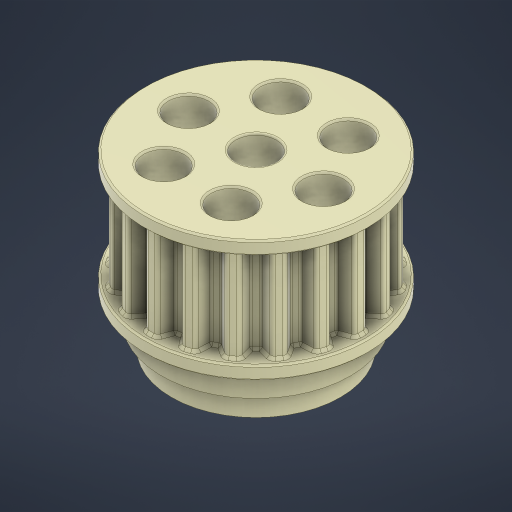
# Autodesk Inventor part: Pulley_Joint1
Saved by Autodesk Inventor 2023 (Build 270158000, 158)
## iProperties
Created: 2023-02-16
Part Number: Pulley_Joint1
Material: ABS Plastic
Document SubType Name: Modeling
Designer: dzw04
Density: 1.06 g/cm^3
Appearance: Smooth - Ash
Author: dzw04
Autodesk Inventor part; units mm, degrees
ref_plane "YZ Plane" through (0, 0, 0) normal (1, 0, 0) x (0, 1, 0)
ref_plane "XZ Plane" through (0, 0, 0) normal (0, 1, 0) x (-1, 0, 0)
ref_plane "XY Plane" through (0, 0, 0) normal (0, 0, 1) x (1, 0, 0)
sketch "Sketch1" plane through (0, 0, 0) normal (0, 1, 0) x (-1, 0, 0)
  circle A0 centre (0, 0) radius 12.5
  dimension "d0" = 25
  constraints: 1 centre point, 1 coincident
  measures "d0" diameter of A0
extrude "Extrusion1" add sketch "Sketch1" along normal blind 3.5
sketch "Sketch2" plane through (0, 3.5, 0) normal (0, 1, 0) x (1, 0, 0)
  circle A0 centre (0, 0) radius 10
  circle A1 centre (-10, 0) radius 1.5
  circle A2 centre (-5, -8.6603) radius 1.5
  circle A3 centre (5, -8.6603) radius 1.5
  circle A4 centre (10, 0) radius 1.5
  circle A5 centre (5, 8.6603) radius 1.5
  circle A6 centre (-5, 8.6603) radius 1.5
  dimension "d3" = 20
  dimension "d4" = 3
  dimension "d7" = 360
  constraints: 6 centre point, 1 coincident, 1 horizontal alignment, 15 other
  measures "d4" diameter of A1
extrude "Extrusion2" cut sketch "Sketch2" against normal through all contours A0 A4 | A0 A4 | A5 A0 | A0 A5 | A3 A0 | A0 A3 | A6 A0 | A0 A6 | A2 A0 | A0 A2 | A1 A0 | A0 A1
sketch "Sketch3" plane through (0, 0, 0) normal (0, -1, 0) x (1, 0, 0)
  line L0 (0, -5.7158) -> (-4.95, -2.8579)
  line L1 (-4.95, -2.8579) -> (-4.95, 2.8579)
  line L2 (-4.95, 2.8579) -> (0, 5.7158)
  line L3 (0, 5.7158) -> (4.95, 2.8579)
  line L4 (4.95, 2.8579) -> (4.95, -2.8579)
  line L5 (4.95, -2.8579) -> (0, -5.7158)
  point P0 (0, 0)
  point P1 (0, 0)
  dimension "d11" = 4.95
  constraints: 12 end point, 1 coincident, 13 other
  measures "d11" distance from line of L5 point (0, 0)
extrude "Extrusion3" add sketch "Sketch3" along normal blind 1.75
chamfer "Chamfer1" distance 1 angle 45 6 edges at (4.95, 0, 0) (2.475, 0, 4.2868) (2.475, 0, -4.2868) (-2.475, 0, -4.2868) (-4.95, 0, 0) (-2.475, 0, 4.2868)
sketch "Sketch4" plane through (0, 3.5, 0) normal (0, 1, 0) x (1, 0, 0)
  circle A0 centre (0, 0) radius 14
  circle A1 centre (5, 8.6603) radius 1.5 projected
  circle A2 centre (-5, -8.6603) radius 1.5 projected
  circle A3 centre (-5, 8.6603) radius 1.5 projected
  circle A4 centre (10, 0) radius 1.5 projected
  circle A5 centre (5, -8.6603) radius 1.5 projected
  circle A6 centre (-10, 0) radius 1.5 projected
  circle A7 centre (0, 0) radius 12.5 projected
  dimension "d17" = 28
  constraints: 1 centre point, 1 coincident
  measures "d17" diameter of A0
extrude "Extrusion4" add sketch "Sketch4" along normal blind 6 contours A0 | A7
sketch "Sketch5" plane through (0, 9.5, 0) normal (0, 1, 0) x (1, 0, 0)
  circle A0 centre (0, 0) radius 16.5
  circle A1 centre (0, 0) radius 14
  dimension "d20" = 33
  dimension "d21" = 28
  constraints: 2 centre point, 2 coincident
  measures "d20" diameter of A0
  measures "d21" diameter of A1
extrude "Extrusion5" add sketch "Sketch5" against normal blind 2
sketch "Sketch6" plane through (0, 9.5, 0) normal (0, 1, 0) x (1, 0, 0)
  arc A0 (-1.7917, 13.431) -> (-2.4464, 13.3273) centre (0, 0) ccw
  arc A1 (-2.8316, 13.4718) -> (-2.4464, 13.3273) centre (-2.5186, 13.7208) ccw
  line L0 (-2.8316, 13.4718) -> (-3.774, 14.6565)
  arc A2 (-3.774, 14.6565) -> (-4.4144, 14.8581) centre (-4.2435, 14.2829) ccw
  arc A3 (-4.4144, 14.8581) -> (-5.162, 14.6152) centre (0, 0) ccw
  arc A4 (-5.162, 14.6152) -> (-5.5616, 14.0756) centre (-4.9622, 14.0494) ccw
  line L1 (-5.5616, 14.0756) -> (-5.6277, 12.5633)
  arc A5 (-5.8545, 12.22) -> (-5.6277, 12.5633) centre (-6.0273, 12.5807) ccw
  arc A6 (-5.8545, 12.22) -> (-6.445, 11.9191) centre (0, 0) ccw
  arc A7 (-6.856, 11.9374) -> (-6.445, 11.9191) centre (-6.6353, 12.2709) ccw
  line L2 (-6.856, 11.9374) -> (-8.1183, 12.7729)
  arc A8 (-8.1183, 12.7729) -> (-8.7898, 12.7668) centre (-8.4495, 12.2726) ccw
  arc A9 (-8.7898, 12.7668) -> (-9.4257, 12.3047) centre (0, 0) ccw
  arc A10 (-9.4257, 12.3047) -> (-9.639, 11.668) centre (-9.0609, 11.8284) ccw
  line L3 (-9.639, 11.668) -> (-9.2345, 10.2093)
  arc A11 (-9.3441, 9.8128) -> (-9.2345, 10.2093) centre (-9.6199, 10.1024) ccw
  arc A12 (-9.3441, 9.8128) -> (-9.8128, 9.3441) centre (0, 0) ccw
  arc A13 (-10.2093, 9.2345) -> (-9.8128, 9.3441) centre (-10.1024, 9.6199) ccw
  line L4 (-10.2093, 9.2345) -> (-11.668, 9.639)
  arc A14 (-11.668, 9.639) -> (-12.3047, 9.4257) centre (-11.8284, 9.0609) ccw
  arc A15 (-12.3047, 9.4257) -> (-12.7668, 8.7898) centre (0, 0) ccw
  arc A16 (-12.7668, 8.7898) -> (-12.7729, 8.1183) centre (-12.2726, 8.4495) ccw
  line L5 (-12.7729, 8.1183) -> (-11.9374, 6.856)
  arc A17 (-11.9191, 6.445) -> (-11.9374, 6.856) centre (-12.2709, 6.6353) ccw
  arc A18 (-11.9191, 6.445) -> (-12.22, 5.8545) centre (0, 0) ccw
  arc A19 (-12.5633, 5.6277) -> (-12.22, 5.8545) centre (-12.5807, 6.0273) ccw
  line L6 (-12.5633, 5.6277) -> (-14.0756, 5.5616)
  arc A20 (-14.0756, 5.5616) -> (-14.6152, 5.162) centre (-14.0494, 4.9622) ccw
  arc A21 (-14.6152, 5.162) -> (-14.8581, 4.4144) centre (0, 0) ccw
  arc A22 (-14.8581, 4.4144) -> (-14.6565, 3.774) centre (-14.2829, 4.2435) ccw
  line L7 (-14.6565, 3.774) -> (-13.4718, 2.8316)
  arc A23 (-13.3273, 2.4464) -> (-13.4718, 2.8316) centre (-13.7208, 2.5186) ccw
  arc A24 (-13.3273, 2.4464) -> (-13.431, 1.7917) centre (0, 0) ccw
  arc A25 (-13.6874, 1.47) -> (-13.431, 1.7917) centre (-13.8275, 1.8446) ccw
  line L8 (-13.6874, 1.47) -> (-15.1053, 0.9398)
  arc A26 (-15.1053, 0.9398) -> (-15.495, 0.393) centre (-14.8952, 0.3778) ccw
  arc A27 (-15.495, 0.393) -> (-15.495, -0.393) centre (0, 0) ccw
  arc A28 (-15.495, -0.393) -> (-15.1053, -0.9398) centre (-14.8952, -0.3778) ccw
  line L9 (-15.1053, -0.9398) -> (-13.6874, -1.47)
  arc A29 (-13.431, -1.7917) -> (-13.6874, -1.47) centre (-13.8275, -1.8446) ccw
  arc A30 (-13.431, -1.7917) -> (-13.3273, -2.4464) centre (0, 0) ccw
  arc A31 (-13.4718, -2.8316) -> (-13.3273, -2.4464) centre (-13.7208, -2.5186) ccw
  line L10 (-13.4718, -2.8316) -> (-14.6565, -3.774)
  arc A32 (-14.6565, -3.774) -> (-14.8581, -4.4144) centre (-14.2829, -4.2435) ccw
  arc A33 (-14.8581, -4.4144) -> (-14.6152, -5.162) centre (0, 0) ccw
  arc A34 (-14.6152, -5.162) -> (-14.0756, -5.5616) centre (-14.0494, -4.9622) ccw
  line L11 (-14.0756, -5.5616) -> (-12.5633, -5.6277)
  arc A35 (-12.22, -5.8545) -> (-12.5633, -5.6277) centre (-12.5807, -6.0273) ccw
  arc A36 (-12.22, -5.8545) -> (-11.9191, -6.445) centre (0, 0) ccw
  arc A37 (-11.9374, -6.856) -> (-11.9191, -6.445) centre (-12.2709, -6.6353) ccw
  line L12 (-11.9374, -6.856) -> (-12.7729, -8.1183)
  arc A38 (-12.7729, -8.1183) -> (-12.7668, -8.7898) centre (-12.2726, -8.4495) ccw
  arc A39 (-12.7668, -8.7898) -> (-12.3047, -9.4257) centre (0, 0) ccw
  arc A40 (-12.3047, -9.4257) -> (-11.668, -9.639) centre (-11.8284, -9.0609) ccw
  line L13 (-11.668, -9.639) -> (-10.2093, -9.2345)
  arc A41 (-9.8128, -9.3441) -> (-10.2093, -9.2345) centre (-10.1024, -9.6199) ccw
  arc A42 (-9.8128, -9.3441) -> (-9.3441, -9.8128) centre (0, 0) ccw
  arc A43 (-9.2345, -10.2093) -> (-9.3441, -9.8128) centre (-9.6199, -10.1024) ccw
  line L14 (-9.2345, -10.2093) -> (-9.639, -11.668)
  arc A44 (-9.639, -11.668) -> (-9.4257, -12.3047) centre (-9.0609, -11.8284) ccw
  arc A45 (-9.4257, -12.3047) -> (-8.7898, -12.7668) centre (0, 0) ccw
  arc A46 (-8.7898, -12.7668) -> (-8.1183, -12.7729) centre (-8.4495, -12.2726) ccw
  line L15 (-8.1183, -12.7729) -> (-6.856, -11.9374)
  arc A47 (-6.445, -11.9191) -> (-6.856, -11.9374) centre (-6.6353, -12.2709) ccw
  arc A48 (-6.445, -11.9191) -> (-5.8545, -12.22) centre (0, 0) ccw
  arc A49 (-5.6277, -12.5633) -> (-5.8545, -12.22) centre (-6.0273, -12.5807) ccw
  line L16 (-5.6277, -12.5633) -> (-5.5616, -14.0756)
  arc A50 (-5.5616, -14.0756) -> (-5.162, -14.6152) centre (-4.9622, -14.0494) ccw
  arc A51 (-5.162, -14.6152) -> (-4.4144, -14.8581) centre (0, 0) ccw
  arc A52 (-4.4144, -14.8581) -> (-3.774, -14.6565) centre (-4.2435, -14.2829) ccw
  line L17 (-3.774, -14.6565) -> (-2.8316, -13.4718)
  arc A53 (-2.4464, -13.3273) -> (-2.8316, -13.4718) centre (-2.5186, -13.7208) ccw
  arc A54 (-2.4464, -13.3273) -> (-1.7917, -13.431) centre (0, 0) ccw
  arc A55 (-1.47, -13.6874) -> (-1.7917, -13.431) centre (-1.8446, -13.8275) ccw
  line L18 (-1.47, -13.6874) -> (-0.9398, -15.1053)
  arc A56 (-0.9398, -15.1053) -> (-0.393, -15.495) centre (-0.3778, -14.8952) ccw
  arc A57 (-0.393, -15.495) -> (0.393, -15.495) centre (0, 0) ccw
  arc A58 (0.393, -15.495) -> (0.9398, -15.1053) centre (0.3778, -14.8952) ccw
  line L19 (0.9398, -15.1053) -> (1.47, -13.6874)
  arc A59 (1.7917, -13.431) -> (1.47, -13.6874) centre (1.8446, -13.8275) ccw
  arc A60 (1.7917, -13.431) -> (2.4464, -13.3273) centre (0, 0) ccw
  arc A61 (2.8316, -13.4718) -> (2.4464, -13.3273) centre (2.5186, -13.7208) ccw
  line L20 (2.8316, -13.4718) -> (3.774, -14.6565)
  arc A62 (3.774, -14.6565) -> (4.4144, -14.8581) centre (4.2435, -14.2829) ccw
  arc A63 (4.4144, -14.8581) -> (5.162, -14.6152) centre (0, 0) ccw
  arc A64 (5.162, -14.6152) -> (5.5616, -14.0756) centre (4.9622, -14.0494) ccw
  line L21 (5.5616, -14.0756) -> (5.6277, -12.5633)
  arc A65 (5.8545, -12.22) -> (5.6277, -12.5633) centre (6.0273, -12.5807) ccw
  arc A66 (5.8545, -12.22) -> (6.445, -11.9191) centre (0, 0) ccw
  arc A67 (6.856, -11.9374) -> (6.445, -11.9191) centre (6.6353, -12.2709) ccw
  line L22 (6.856, -11.9374) -> (8.1183, -12.7729)
  arc A68 (8.1183, -12.7729) -> (8.7898, -12.7668) centre (8.4495, -12.2726) ccw
  arc A69 (8.7898, -12.7668) -> (9.4257, -12.3047) centre (0, 0) ccw
  arc A70 (9.4257, -12.3047) -> (9.639, -11.668) centre (9.0609, -11.8284) ccw
  line L23 (9.639, -11.668) -> (9.2345, -10.2093)
  arc A71 (9.3441, -9.8128) -> (9.2345, -10.2093) centre (9.6199, -10.1024) ccw
  arc A72 (9.3441, -9.8128) -> (9.8128, -9.3441) centre (0, 0) ccw
  arc A73 (10.2093, -9.2345) -> (9.8128, -9.3441) centre (10.1024, -9.6199) ccw
  line L24 (10.2093, -9.2345) -> (11.668, -9.639)
  arc A74 (11.668, -9.639) -> (12.3047, -9.4257) centre (11.8284, -9.0609) ccw
  arc A75 (12.3047, -9.4257) -> (12.7668, -8.7898) centre (0, 0) ccw
  arc A76 (12.7668, -8.7898) -> (12.7729, -8.1183) centre (12.2726, -8.4495) ccw
  line L25 (12.7729, -8.1183) -> (11.9374, -6.856)
  arc A77 (11.9191, -6.445) -> (11.9374, -6.856) centre (12.2709, -6.6353) ccw
  arc A78 (11.9191, -6.445) -> (12.22, -5.8545) centre (0, 0) ccw
  arc A79 (12.5633, -5.6277) -> (12.22, -5.8545) centre (12.5807, -6.0273) ccw
  line L26 (12.5633, -5.6277) -> (14.0756, -5.5616)
  arc A80 (14.0756, -5.5616) -> (14.6152, -5.162) centre (14.0494, -4.9622) ccw
  arc A81 (14.6152, -5.162) -> (14.8581, -4.4144) centre (0, 0) ccw
  arc A82 (14.8581, -4.4144) -> (14.6565, -3.774) centre (14.2829, -4.2435) ccw
  line L27 (14.6565, -3.774) -> (13.4718, -2.8316)
  arc A83 (13.3273, -2.4464) -> (13.4718, -2.8316) centre (13.7208, -2.5186) ccw
  arc A84 (13.3273, -2.4464) -> (13.431, -1.7917) centre (0, 0) ccw
  arc A85 (13.6874, -1.47) -> (13.431, -1.7917) centre (13.8275, -1.8446) ccw
  line L28 (13.6874, -1.47) -> (15.1053, -0.9398)
  arc A86 (15.1053, -0.9398) -> (15.495, -0.393) centre (14.8952, -0.3778) ccw
  arc A87 (15.495, -0.393) -> (15.495, 0.393) centre (0, 0) ccw
  arc A88 (15.495, 0.393) -> (15.1053, 0.9398) centre (14.8952, 0.3778) ccw
  line L29 (15.1053, 0.9398) -> (13.6874, 1.47)
  arc A89 (13.431, 1.7917) -> (13.6874, 1.47) centre (13.8275, 1.8446) ccw
  arc A90 (13.431, 1.7917) -> (13.3273, 2.4464) centre (0, 0) ccw
  arc A91 (13.4718, 2.8316) -> (13.3273, 2.4464) centre (13.7208, 2.5186) ccw
  line L30 (13.4718, 2.8316) -> (14.6565, 3.774)
  arc A92 (14.6565, 3.774) -> (14.8581, 4.4144) centre (14.2829, 4.2435) ccw
  arc A93 (14.8581, 4.4144) -> (14.6152, 5.162) centre (0, 0) ccw
  arc A94 (14.6152, 5.162) -> (14.0756, 5.5616) centre (14.0494, 4.9622) ccw
  line L31 (14.0756, 5.5616) -> (12.5633, 5.6277)
  arc A95 (12.22, 5.8545) -> (12.5633, 5.6277) centre (12.5807, 6.0273) ccw
  arc A96 (12.22, 5.8545) -> (11.9191, 6.445) centre (0, 0) ccw
  arc A97 (11.9374, 6.856) -> (11.9191, 6.445) centre (12.2709, 6.6353) ccw
  line L32 (11.9374, 6.856) -> (12.7729, 8.1183)
  arc A98 (12.7729, 8.1183) -> (12.7668, 8.7898) centre (12.2726, 8.4495) ccw
  arc A99 (12.7668, 8.7898) -> (12.3047, 9.4257) centre (0, 0) ccw
  arc A100 (12.3047, 9.4257) -> (11.668, 9.639) centre (11.8284, 9.0609) ccw
  line L33 (11.668, 9.639) -> (10.2093, 9.2345)
  arc A101 (9.8128, 9.3441) -> (10.2093, 9.2345) centre (10.1024, 9.6199) ccw
  arc A102 (9.8128, 9.3441) -> (9.3441, 9.8128) centre (0, 0) ccw
  arc A103 (9.2345, 10.2093) -> (9.3441, 9.8128) centre (9.6199, 10.1024) ccw
  line L34 (9.2345, 10.2093) -> (9.639, 11.668)
  arc A104 (9.639, 11.668) -> (9.4257, 12.3047) centre (9.0609, 11.8284) ccw
  arc A105 (9.4257, 12.3047) -> (8.7898, 12.7668) centre (0, 0) ccw
  arc A106 (8.7898, 12.7668) -> (8.1183, 12.7729) centre (8.4495, 12.2726) ccw
  line L35 (8.1183, 12.7729) -> (6.856, 11.9374)
  arc A107 (6.445, 11.9191) -> (6.856, 11.9374) centre (6.6353, 12.2709) ccw
  arc A108 (6.445, 11.9191) -> (5.8545, 12.22) centre (0, 0) ccw
  arc A109 (5.6277, 12.5633) -> (5.8545, 12.22) centre (6.0273, 12.5807) ccw
  line L36 (5.6277, 12.5633) -> (5.5616, 14.0756)
  arc A110 (5.5616, 14.0756) -> (5.162, 14.6152) centre (4.9622, 14.0494) ccw
  arc A111 (5.162, 14.6152) -> (4.4144, 14.8581) centre (0, 0) ccw
  arc A112 (4.4144, 14.8581) -> (3.774, 14.6565) centre (4.2435, 14.2829) ccw
  line L37 (3.774, 14.6565) -> (2.8316, 13.4718)
  arc A113 (2.4464, 13.3273) -> (2.8316, 13.4718) centre (2.5186, 13.7208) ccw
  arc A114 (2.4464, 13.3273) -> (1.7917, 13.431) centre (0, 0) ccw
  arc A115 (1.47, 13.6874) -> (1.7917, 13.431) centre (1.8446, 13.8275) ccw
  line L38 (1.47, 13.6874) -> (0.9398, 15.1053)
  arc A116 (0.9398, 15.1053) -> (0.393, 15.495) centre (0.3778, 14.8952) ccw
  arc A117 (0.393, 15.495) -> (-0.393, 15.495) centre (0, 0) ccw
  arc A118 (-0.393, 15.495) -> (-0.9398, 15.1053) centre (-0.3778, 14.8952) ccw
  line L39 (-0.9398, 15.1053) -> (-1.47, 13.6874)
  arc A119 (-1.7917, 13.431) -> (-1.47, 13.6874) centre (-1.8446, 13.8275) ccw
  circle A120 centre (0, 0) radius 17.75
  circle A121 centre (0, 0) radius 16.5 projected
  circle A122 centre (-10, 0) radius 1.5 projected
  circle A123 centre (5, -8.6603) radius 1.5 projected
  circle A124 centre (10, 0) radius 1.5 projected
  circle A125 centre (-5, 8.6603) radius 1.5 projected
  circle A126 centre (-5, -8.6603) radius 1.5 projected
  circle A127 centre (5, 8.6603) radius 1.5 projected
  point P0 (1.47, 13.6874)
  point P1 (0.393, 15.495)
  point P2 (-0.393, 15.495)
  point P3 (-0.9398, 15.1053)
  point P4 (-1.7917, 13.431)
  point P5 (-2.4464, 13.3273)
  point P6 (-2.8316, 13.4718)
  point P7 (-4.4144, 14.8581)
  point P8 (-5.162, 14.6152)
  point P9 (-5.5616, 14.0756)
  point P10 (-5.8545, 12.22)
  point P11 (-6.445, 11.9191)
  point P12 (-6.856, 11.9374)
  point P13 (-8.7898, 12.7668)
  point P14 (-9.4257, 12.3047)
  point P15 (-9.3441, 9.8128)
  point P16 (-9.8128, 9.3441)
  point P17 (-10.2093, 9.2345)
  point P18 (-12.3047, 9.4257)
  point P19 (-12.7668, 8.7898)
  point P20 (-12.7729, 8.1183)
  point P21 (-11.9191, 6.445)
  point P22 (-12.22, 5.8545)
  point P23 (-12.5633, 5.6277)
  point P24 (-14.8581, 4.4144)
  point P25 (-14.6565, 3.774)
  point P26 (-13.3273, 2.4464)
  point P27 (-13.431, 1.7917)
  point P28 (-13.6874, 1.47)
  point P29 (-15.495, 0.393)
  point P30 (-15.495, -0.393)
  point P31 (-15.1053, -0.9398)
  point P32 (-13.3273, -2.4464)
  point P33 (-13.4718, -2.8316)
  point P34 (-14.8581, -4.4144)
  point P35 (-14.6152, -5.162)
  point P36 (-14.0756, -5.5616)
  point P37 (-12.22, -5.8545)
  point P38 (-11.9191, -6.445)
  point P39 (-12.7668, -8.7898)
  point P40 (-12.3047, -9.4257)
  point P41 (-9.8128, -9.3441)
  point P42 (-9.3441, -9.8128)
  point P43 (-9.2345, -10.2093)
  point P44 (-9.4257, -12.3047)
  point P45 (-8.7898, -12.7668)
  point P46 (-6.445, -11.9191)
  point P47 (-5.8545, -12.22)
  point P48 (-5.162, -14.6152)
  point P49 (-4.4144, -14.8581)
  point P50 (-2.4464, -13.3273)
  point P51 (-1.7917, -13.431)
  point P52 (-1.47, -13.6874)
  point P53 (-0.393, -15.495)
  point P54 (0.393, -15.495)
  point P55 (0.9398, -15.1053)
  point P56 (1.7917, -13.431)
  point P57 (2.4464, -13.3273)
  point P58 (2.8316, -13.4718)
  point P59 (4.4144, -14.8581)
  point P60 (5.162, -14.6152)
  point P61 (5.8545, -12.22)
  point P62 (6.445, -11.9191)
  point P63 (6.856, -11.9374)
  point P64 (8.7898, -12.7668)
  point P65 (9.4257, -12.3047)
  point P66 (9.3441, -9.8128)
  point P67 (9.8128, -9.3441)
  point P68 (10.2093, -9.2345)
  point P69 (12.3047, -9.4257)
  point P70 (12.7668, -8.7898)
  point P71 (12.7729, -8.1183)
  point P72 (11.9191, -6.445)
  point P73 (12.22, -5.8545)
  point P74 (12.5633, -5.6277)
  point P75 (14.6152, -5.162)
  point P76 (14.8581, -4.4144)
  point P77 (14.6565, -3.774)
  point P78 (13.3273, -2.4464)
  point P79 (13.431, -1.7917)
  point P80 (13.6874, -1.47)
  point P81 (15.495, -0.393)
  point P82 (15.495, 0.393)
  point P83 (15.1053, 0.9398)
  point P84 (13.3273, 2.4464)
  point P85 (13.4718, 2.8316)
  point P86 (14.8581, 4.4144)
  point P87 (14.6152, 5.162)
  point P88 (14.0756, 5.5616)
  point P89 (12.22, 5.8545)
  point P90 (11.9191, 6.445)
  point P91 (11.9374, 6.856)
  point P92 (12.7668, 8.7898)
  point P93 (12.3047, 9.4257)
  point P94 (9.8128, 9.3441)
  point P95 (9.3441, 9.8128)
  point P96 (9.2345, 10.2093)
  point P97 (9.4257, 12.3047)
  point P98 (8.7898, 12.7668)
  point P99 (8.1183, 12.7729)
  point P100 (6.445, 11.9191)
  point P101 (5.8545, 12.22)
  point P102 (5.6277, 12.5633)
  point P103 (5.162, 14.6152)
  point P104 (4.4144, 14.8581)
  point P105 (3.774, 14.6565)
  point P106 (2.4464, 13.3273)
  point P107 (1.7917, 13.431)
  constraints: 240 point on circle, 121 centre point, 80 end point
extrude "Extrusion6" add sketch "Sketch6" along normal blind 14 contours A119 L39 A118 A117 A116 L38 A115 A114 A113 L37 A112 A111 A110 L36 A109 A108 A107 L35 A106 A105 A104 L34 A103 A102 A101 L33 A100 A99 A98 L32 A97 A96 A95 L31 A94 A93 A92 L30 A91 A90 A89 L29 A88 A87 A86 L28 A85 A84 A83 L27 A82 A81 A80 L26 A79 A78 A77 L25 A76 A75 A74 L24 A73 A72 A71 L23 A70 A69 A68 L22 A67 A66 A65 L21 A64 A63 A62 L20 A61 A60 A59 L19 A58 A57 A56 L18 A55 A54 A53 L17 A52 A51 A50 L16 A49 A48 A47 L15 A46 A45 A44 L14 A43 A42 A41 L13 A40 A39 A38 L12 A37 A36 A35 L11 A34 A33 A32 L10 A31 A30 A29 L9 A28 A27 A26 L8 A25 A24 A23 L7 A22 A21 A20 L6 A19 A18 A17 L5 A16 A15 A14 L4 A13 A12 A11 L3 A10 A9 A8 L2 A7 A6 A5 L1 A4 A3 A2 L0 A1 A0
sketch "Sketch7" plane through (0, 23.5, 0) normal (0, 1, 0) x (1, 0, 0)
  circle A0 centre (0, 0) radius 16.5
  arc A1 (0.9398, 15.1053) -> (0.393, 15.495) centre (0.3778, 14.8952) ccw projected
  arc A2 (0.393, 15.495) -> (-0.393, 15.495) centre (0, 0) ccw projected
  arc A3 (-0.393, 15.495) -> (-0.9398, 15.1053) centre (-0.3778, 14.8952) ccw projected
  line L0 (-0.9398, 15.1053) -> (-1.47, 13.6874) projected
  arc A4 (-1.7917, 13.431) -> (-1.47, 13.6874) centre (-1.8446, 13.8275) ccw projected
  arc A5 (-1.7917, 13.431) -> (-2.4464, 13.3273) centre (0, 0) ccw projected
  arc A6 (-2.8316, 13.4718) -> (-2.4464, 13.3273) centre (-2.5186, 13.7208) ccw projected
  line L1 (-2.8316, 13.4718) -> (-3.774, 14.6565) projected
  arc A7 (-3.774, 14.6565) -> (-4.4144, 14.8581) centre (-4.2435, 14.2829) ccw projected
  arc A8 (-4.4144, 14.8581) -> (-5.162, 14.6152) centre (0, 0) ccw projected
  arc A9 (-5.162, 14.6152) -> (-5.5616, 14.0756) centre (-4.9622, 14.0494) ccw projected
  line L2 (-5.5616, 14.0756) -> (-5.6277, 12.5633) projected
  arc A10 (-5.8545, 12.22) -> (-5.6277, 12.5633) centre (-6.0273, 12.5807) ccw projected
  arc A11 (-5.8545, 12.22) -> (-6.445, 11.9191) centre (0, 0) ccw projected
  arc A12 (-6.856, 11.9374) -> (-6.445, 11.9191) centre (-6.6353, 12.2709) ccw projected
  line L3 (-6.856, 11.9374) -> (-8.1183, 12.7729) projected
  arc A13 (-8.1183, 12.7729) -> (-8.7898, 12.7668) centre (-8.4495, 12.2726) ccw projected
  arc A14 (-8.7898, 12.7668) -> (-9.4257, 12.3047) centre (0, 0) ccw projected
  arc A15 (-9.4257, 12.3047) -> (-9.639, 11.668) centre (-9.0609, 11.8284) ccw projected
  line L4 (-9.639, 11.668) -> (-9.2345, 10.2093) projected
  arc A16 (-9.3441, 9.8128) -> (-9.2345, 10.2093) centre (-9.6199, 10.1024) ccw projected
  arc A17 (-9.3441, 9.8128) -> (-9.8128, 9.3441) centre (0, 0) ccw projected
  arc A18 (-10.2093, 9.2345) -> (-9.8128, 9.3441) centre (-10.1024, 9.6199) ccw projected
  line L5 (-10.2093, 9.2345) -> (-11.668, 9.639) projected
  arc A19 (-11.668, 9.639) -> (-12.3047, 9.4257) centre (-11.8284, 9.0609) ccw projected
  arc A20 (-12.3047, 9.4257) -> (-12.7668, 8.7898) centre (0, 0) ccw projected
  arc A21 (-12.7668, 8.7898) -> (-12.7729, 8.1183) centre (-12.2726, 8.4495) ccw projected
  line L6 (-12.7729, 8.1183) -> (-11.9374, 6.856) projected
  arc A22 (-11.9191, 6.445) -> (-11.9374, 6.856) centre (-12.2709, 6.6353) ccw projected
  arc A23 (-11.9191, 6.445) -> (-12.22, 5.8545) centre (0, 0) ccw projected
  arc A24 (-12.5633, 5.6277) -> (-12.22, 5.8545) centre (-12.5807, 6.0273) ccw projected
  line L7 (-12.5633, 5.6277) -> (-14.0756, 5.5616) projected
  arc A25 (-14.0756, 5.5616) -> (-14.6152, 5.162) centre (-14.0494, 4.9622) ccw projected
  arc A26 (-14.6152, 5.162) -> (-14.8581, 4.4144) centre (0, 0) ccw projected
  arc A27 (-14.8581, 4.4144) -> (-14.6565, 3.774) centre (-14.2829, 4.2435) ccw projected
  line L8 (-14.6565, 3.774) -> (-13.4718, 2.8316) projected
  arc A28 (-13.3273, 2.4464) -> (-13.4718, 2.8316) centre (-13.7208, 2.5186) ccw projected
  arc A29 (-13.3273, 2.4464) -> (-13.431, 1.7917) centre (0, 0) ccw projected
  arc A30 (-13.6874, 1.47) -> (-13.431, 1.7917) centre (-13.8275, 1.8446) ccw projected
  line L9 (-13.6874, 1.47) -> (-15.1053, 0.9398) projected
  arc A31 (-15.1053, 0.9398) -> (-15.495, 0.393) centre (-14.8952, 0.3778) ccw projected
  arc A32 (-15.495, 0.393) -> (-15.495, -0.393) centre (0, 0) ccw projected
  arc A33 (-15.495, -0.393) -> (-15.1053, -0.9398) centre (-14.8952, -0.3778) ccw projected
  line L10 (-15.1053, -0.9398) -> (-13.6874, -1.47) projected
  arc A34 (-13.431, -1.7917) -> (-13.6874, -1.47) centre (-13.8275, -1.8446) ccw projected
  arc A35 (-13.431, -1.7917) -> (-13.3273, -2.4464) centre (0, 0) ccw projected
  arc A36 (-13.4718, -2.8316) -> (-13.3273, -2.4464) centre (-13.7208, -2.5186) ccw projected
  line L11 (-13.4718, -2.8316) -> (-14.6565, -3.774) projected
  arc A37 (-14.6565, -3.774) -> (-14.8581, -4.4144) centre (-14.2829, -4.2435) ccw projected
  arc A38 (-14.8581, -4.4144) -> (-14.6152, -5.162) centre (0, 0) ccw projected
  arc A39 (-14.6152, -5.162) -> (-14.0756, -5.5616) centre (-14.0494, -4.9622) ccw projected
  line L12 (-14.0756, -5.5616) -> (-12.5633, -5.6277) projected
  arc A40 (-12.22, -5.8545) -> (-12.5633, -5.6277) centre (-12.5807, -6.0273) ccw projected
  arc A41 (-12.22, -5.8545) -> (-11.9191, -6.445) centre (0, 0) ccw projected
  arc A42 (-11.9374, -6.856) -> (-11.9191, -6.445) centre (-12.2709, -6.6353) ccw projected
  line L13 (-11.9374, -6.856) -> (-12.7729, -8.1183) projected
  arc A43 (-12.7729, -8.1183) -> (-12.7668, -8.7898) centre (-12.2726, -8.4495) ccw projected
  arc A44 (-12.7668, -8.7898) -> (-12.3047, -9.4257) centre (0, 0) ccw projected
  arc A45 (-12.3047, -9.4257) -> (-11.668, -9.639) centre (-11.8284, -9.0609) ccw projected
  line L14 (-11.668, -9.639) -> (-10.2093, -9.2345) projected
  arc A46 (-9.8128, -9.3441) -> (-10.2093, -9.2345) centre (-10.1024, -9.6199) ccw projected
  arc A47 (-9.8128, -9.3441) -> (-9.3441, -9.8128) centre (0, 0) ccw projected
  arc A48 (-9.2345, -10.2093) -> (-9.3441, -9.8128) centre (-9.6199, -10.1024) ccw projected
  line L15 (-9.2345, -10.2093) -> (-9.639, -11.668) projected
  arc A49 (-9.639, -11.668) -> (-9.4257, -12.3047) centre (-9.0609, -11.8284) ccw projected
  arc A50 (-9.4257, -12.3047) -> (-8.7898, -12.7668) centre (0, 0) ccw projected
  arc A51 (-8.7898, -12.7668) -> (-8.1183, -12.7729) centre (-8.4495, -12.2726) ccw projected
  line L16 (-8.1183, -12.7729) -> (-6.856, -11.9374) projected
  arc A52 (-6.445, -11.9191) -> (-6.856, -11.9374) centre (-6.6353, -12.2709) ccw projected
  arc A53 (-6.445, -11.9191) -> (-5.8545, -12.22) centre (0, 0) ccw projected
  arc A54 (-5.6277, -12.5633) -> (-5.8545, -12.22) centre (-6.0273, -12.5807) ccw projected
  line L17 (-5.6277, -12.5633) -> (-5.5616, -14.0756) projected
  arc A55 (-5.5616, -14.0756) -> (-5.162, -14.6152) centre (-4.9622, -14.0494) ccw projected
  arc A56 (-5.162, -14.6152) -> (-4.4144, -14.8581) centre (0, 0) ccw projected
  arc A57 (-4.4144, -14.8581) -> (-3.774, -14.6565) centre (-4.2435, -14.2829) ccw projected
  line L18 (-3.774, -14.6565) -> (-2.8316, -13.4718) projected
  arc A58 (-2.4464, -13.3273) -> (-2.8316, -13.4718) centre (-2.5186, -13.7208) ccw projected
  arc A59 (-2.4464, -13.3273) -> (-1.7917, -13.431) centre (0, 0) ccw projected
  arc A60 (-1.47, -13.6874) -> (-1.7917, -13.431) centre (-1.8446, -13.8275) ccw projected
  line L19 (-1.47, -13.6874) -> (-0.9398, -15.1053) projected
  arc A61 (-0.9398, -15.1053) -> (-0.393, -15.495) centre (-0.3778, -14.8952) ccw projected
  arc A62 (-0.393, -15.495) -> (0.393, -15.495) centre (0, 0) ccw projected
  arc A63 (0.393, -15.495) -> (0.9398, -15.1053) centre (0.3778, -14.8952) ccw projected
  line L20 (0.9398, -15.1053) -> (1.47, -13.6874) projected
  arc A64 (1.7917, -13.431) -> (1.47, -13.6874) centre (1.8446, -13.8275) ccw projected
  arc A65 (1.7917, -13.431) -> (2.4464, -13.3273) centre (0, 0) ccw projected
  arc A66 (2.8316, -13.4718) -> (2.4464, -13.3273) centre (2.5186, -13.7208) ccw projected
  line L21 (2.8316, -13.4718) -> (3.774, -14.6565) projected
  arc A67 (3.774, -14.6565) -> (4.4144, -14.8581) centre (4.2435, -14.2829) ccw projected
  arc A68 (4.4144, -14.8581) -> (5.162, -14.6152) centre (0, 0) ccw projected
  arc A69 (5.162, -14.6152) -> (5.5616, -14.0756) centre (4.9622, -14.0494) ccw projected
  line L22 (5.5616, -14.0756) -> (5.6277, -12.5633) projected
  arc A70 (5.8545, -12.22) -> (5.6277, -12.5633) centre (6.0273, -12.5807) ccw projected
  arc A71 (5.8545, -12.22) -> (6.445, -11.9191) centre (0, 0) ccw projected
  arc A72 (6.856, -11.9374) -> (6.445, -11.9191) centre (6.6353, -12.2709) ccw projected
  line L23 (6.856, -11.9374) -> (8.1183, -12.7729) projected
  arc A73 (8.1183, -12.7729) -> (8.7898, -12.7668) centre (8.4495, -12.2726) ccw projected
  arc A74 (8.7898, -12.7668) -> (9.4257, -12.3047) centre (0, 0) ccw projected
  arc A75 (9.4257, -12.3047) -> (9.639, -11.668) centre (9.0609, -11.8284) ccw projected
  line L24 (9.639, -11.668) -> (9.2345, -10.2093) projected
  arc A76 (9.3441, -9.8128) -> (9.2345, -10.2093) centre (9.6199, -10.1024) ccw projected
  arc A77 (9.3441, -9.8128) -> (9.8128, -9.3441) centre (0, 0) ccw projected
  arc A78 (10.2093, -9.2345) -> (9.8128, -9.3441) centre (10.1024, -9.6199) ccw projected
  line L25 (10.2093, -9.2345) -> (11.668, -9.639) projected
  arc A79 (11.668, -9.639) -> (12.3047, -9.4257) centre (11.8284, -9.0609) ccw projected
  arc A80 (12.3047, -9.4257) -> (12.7668, -8.7898) centre (0, 0) ccw projected
  arc A81 (12.7668, -8.7898) -> (12.7729, -8.1183) centre (12.2726, -8.4495) ccw projected
  line L26 (12.7729, -8.1183) -> (11.9374, -6.856) projected
  arc A82 (11.9191, -6.445) -> (11.9374, -6.856) centre (12.2709, -6.6353) ccw projected
  arc A83 (11.9191, -6.445) -> (12.22, -5.8545) centre (0, 0) ccw projected
  arc A84 (12.5633, -5.6277) -> (12.22, -5.8545) centre (12.5807, -6.0273) ccw projected
  line L27 (12.5633, -5.6277) -> (14.0756, -5.5616) projected
  arc A85 (14.0756, -5.5616) -> (14.6152, -5.162) centre (14.0494, -4.9622) ccw projected
  arc A86 (14.6152, -5.162) -> (14.8581, -4.4144) centre (0, 0) ccw projected
  arc A87 (14.8581, -4.4144) -> (14.6565, -3.774) centre (14.2829, -4.2435) ccw projected
  line L28 (14.6565, -3.774) -> (13.4718, -2.8316) projected
  arc A88 (13.3273, -2.4464) -> (13.4718, -2.8316) centre (13.7208, -2.5186) ccw projected
  arc A89 (13.3273, -2.4464) -> (13.431, -1.7917) centre (0, 0) ccw projected
  arc A90 (13.6874, -1.47) -> (13.431, -1.7917) centre (13.8275, -1.8446) ccw projected
  line L29 (13.6874, -1.47) -> (15.1053, -0.9398) projected
  arc A91 (15.1053, -0.9398) -> (15.495, -0.393) centre (14.8952, -0.3778) ccw projected
  arc A92 (15.495, -0.393) -> (15.495, 0.393) centre (0, 0) ccw projected
  arc A93 (15.495, 0.393) -> (15.1053, 0.9398) centre (14.8952, 0.3778) ccw projected
  line L30 (15.1053, 0.9398) -> (13.6874, 1.47) projected
  arc A94 (13.431, 1.7917) -> (13.6874, 1.47) centre (13.8275, 1.8446) ccw projected
  arc A95 (13.431, 1.7917) -> (13.3273, 2.4464) centre (0, 0) ccw projected
  arc A96 (13.4718, 2.8316) -> (13.3273, 2.4464) centre (13.7208, 2.5186) ccw projected
  line L31 (13.4718, 2.8316) -> (14.6565, 3.774) projected
  arc A97 (14.6565, 3.774) -> (14.8581, 4.4144) centre (14.2829, 4.2435) ccw projected
  arc A98 (14.8581, 4.4144) -> (14.6152, 5.162) centre (0, 0) ccw projected
  arc A99 (14.6152, 5.162) -> (14.0756, 5.5616) centre (14.0494, 4.9622) ccw projected
  line L32 (14.0756, 5.5616) -> (12.5633, 5.6277) projected
  arc A100 (12.22, 5.8545) -> (12.5633, 5.6277) centre (12.5807, 6.0273) ccw projected
  arc A101 (12.22, 5.8545) -> (11.9191, 6.445) centre (0, 0) ccw projected
  arc A102 (11.9374, 6.856) -> (11.9191, 6.445) centre (12.2709, 6.6353) ccw projected
  line L33 (11.9374, 6.856) -> (12.7729, 8.1183) projected
  arc A103 (12.7729, 8.1183) -> (12.7668, 8.7898) centre (12.2726, 8.4495) ccw projected
  arc A104 (12.7668, 8.7898) -> (12.3047, 9.4257) centre (0, 0) ccw projected
  arc A105 (12.3047, 9.4257) -> (11.668, 9.639) centre (11.8284, 9.0609) ccw projected
  line L34 (11.668, 9.639) -> (10.2093, 9.2345) projected
  arc A106 (9.8128, 9.3441) -> (10.2093, 9.2345) centre (10.1024, 9.6199) ccw projected
  arc A107 (9.8128, 9.3441) -> (9.3441, 9.8128) centre (0, 0) ccw projected
  arc A108 (9.2345, 10.2093) -> (9.3441, 9.8128) centre (9.6199, 10.1024) ccw projected
  line L35 (9.2345, 10.2093) -> (9.639, 11.668) projected
  arc A109 (9.639, 11.668) -> (9.4257, 12.3047) centre (9.0609, 11.8284) ccw projected
  arc A110 (9.4257, 12.3047) -> (8.7898, 12.7668) centre (0, 0) ccw projected
  arc A111 (8.7898, 12.7668) -> (8.1183, 12.7729) centre (8.4495, 12.2726) ccw projected
  line L36 (8.1183, 12.7729) -> (6.856, 11.9374) projected
  arc A112 (6.445, 11.9191) -> (6.856, 11.9374) centre (6.6353, 12.2709) ccw projected
  arc A113 (6.445, 11.9191) -> (5.8545, 12.22) centre (0, 0) ccw projected
  arc A114 (5.6277, 12.5633) -> (5.8545, 12.22) centre (6.0273, 12.5807) ccw projected
  line L37 (5.6277, 12.5633) -> (5.5616, 14.0756) projected
  arc A115 (5.5616, 14.0756) -> (5.162, 14.6152) centre (4.9622, 14.0494) ccw projected
  arc A116 (5.162, 14.6152) -> (4.4144, 14.8581) centre (0, 0) ccw projected
  arc A117 (4.4144, 14.8581) -> (3.774, 14.6565) centre (4.2435, 14.2829) ccw projected
  line L38 (3.774, 14.6565) -> (2.8316, 13.4718) projected
  arc A118 (2.4464, 13.3273) -> (2.8316, 13.4718) centre (2.5186, 13.7208) ccw projected
  arc A119 (2.4464, 13.3273) -> (1.7917, 13.431) centre (0, 0) ccw projected
  arc A120 (1.47, 13.6874) -> (1.7917, 13.431) centre (1.8446, 13.8275) ccw projected
  line L39 (1.47, 13.6874) -> (0.9398, 15.1053) projected
  circle A121 centre (5, 8.6603) radius 1.5 projected
  circle A122 centre (-5, -8.6603) radius 1.5 projected
  circle A123 centre (-5, 8.6603) radius 1.5 projected
  circle A124 centre (10, 0) radius 1.5 projected
  circle A125 centre (5, -8.6603) radius 1.5 projected
  circle A126 centre (-10, 0) radius 1.5 projected
  dimension "d26" = 33
  constraints: 1 centre point, 1 coincident
  measures "d26" diameter of A0
extrude "Extrusion7" add sketch "Sketch7" along normal blind 2 contours A0 | L39 A120 A119 A118 L38 A117 A116 A115 L37 A114 A113 A112 L36 A111 A110 A109 L35 A108 A107 A106 L34 A105 A104 A103 L33 A102 A101 A100 L32 A99 A98 A97 L31 A96 A95 A94 L30 A93 A92 A91 L29 A90 A89 A88 L28 A87 A86 A85 L27 A84 A83 A82 L26 A81 A80 A79 L25 A78 A77 A76 L24 A75 A74 A73 L23 A72 A71 A70 L22 A69 A68 A67 L21 A66 A65 A64 L20 A63 A62 A61 L19 A60 A59 A58 L18 A57 A56 A55 L17 A54 A53 A52 L16 A51 A50 A49 L15 A48 A47 A46 L14 A45 A44 A43 L13 A42 A41 A40 L12 A39 A38 A37 L11 A36 A35 A34 L10 A33 A32 A31 L9 A30 A29 A28 L8 A27 A26 A25 L7 A24 A23 A22 L6 A21 A20 A19 L5 A18 A17 A16 L4 A15 A14 A13 L3 A12 A11 A10 L2 A9 A8 A7 L1 A6 A5 A4 L0 A3 A2 A1
sketch "Sketch8" plane through (0, 25.5, 0) normal (0, 1, 0) x (1, 0, 0)
  circle A0 centre (5, -8.6603) radius 1.5 projected
  circle A1 centre (5, -8.6603) radius 3
  circle A2 centre (-5, -8.6603) radius 1.5 projected
  circle A3 centre (-5, -8.6603) radius 3
  circle A4 centre (-10, 0) radius 1.5 projected
  circle A5 centre (-10, 0) radius 3
  circle A6 centre (-5, 8.6603) radius 1.5 projected
  circle A7 centre (-5, 8.6603) radius 3
  circle A8 centre (5, 8.6603) radius 1.5 projected
  circle A9 centre (5, 8.6603) radius 3
  circle A10 centre (10, 0) radius 1.5 projected
  circle A11 centre (10, 0) radius 3
  point P0 (0, 0)
  dimension "d29" = 6
  dimension "d30" = 6
  dimension "d31" = 6
  dimension "d32" = 6
  dimension "d33" = 6
  dimension "d34" = 6
  constraints: 6 centre point, 6 coincident
  measures "d29" diameter of A1
  measures "d30" diameter of A3
  measures "d31" diameter of A5
  measures "d32" diameter of A7
  measures "d33" diameter of A9
  measures "d34" diameter of A11
extrude "Extrusion8" cut sketch "Sketch8" against normal blind 5
chamfer "Chamfer2" distance 0.25 angle 45 10 edges at (-16.5, 25.5, 0) (-8, 25.5, -8.6603) (-13, 25.5, 0) (-8, 25.5, 8.6603) (2, 25.5, 8.6603) (7, 25.5, 0) (2, 25.5, -8.6603) (-16.5, 23.5, 0) (-16.5, 9.5, 0) (-16.5, 7.5, 0)
chamfer "Chamfer3" distance 0.4 angle 45 260 edges at (9.5813, 23.5, -9.5813) (9.2344, 23.5, -9.9959) (9.4368, 23.5, -10.9387) (9.6298, 23.5, -12.019) (9.1107, 23.5, -12.5398) (8.455, 23.5, -12.8725) (7.4872, 23.5, -12.3551) (6.653, 23.5, -11.8713) (6.1516, 23.5, -12.0731) (5.6935, 23.5, -12.3602) (5.5947, 23.5, -13.3194) (5.4444, 23.5, -14.4065) (4.7898, 23.5, -14.7414) (4.0633, 23.5, -14.8552) (3.3028, 23.5, -14.0641) (2.659, 23.5, -13.3462) (2.1197, 23.5, -13.3832) (1.5954, 23.5, -13.5147) (1.2049, 23.5, -14.3964) (0.7261, 23.5, -15.3838) (0, 23.5, -15.5) (-0.7261, 23.5, -15.3838) (-1.2049, 23.5, -14.3964) (-1.5954, 23.5, -13.5147) (-2.1197, 23.5, -13.3832) (-2.659, 23.5, -13.3462) (-3.3028, 23.5, -14.0641) (-4.0633, 23.5, -14.8552) (-4.7898, 23.5, -14.7414) (-5.4444, 23.5, -14.4065) (-5.5947, 23.5, -13.3194) (-5.6935, 23.5, -12.3602) (-6.1516, 23.5, -12.0731) (-6.653, 23.5, -11.8713) (-7.4872, 23.5, -12.3551) (-8.455, 23.5, -12.8725) (-9.1107, 23.5, -12.5398) (-9.6298, 23.5, -12.019) (-9.4368, 23.5, -10.9387) (-9.2344, 23.5, -9.9959) (-9.5813, 23.5, -9.5813) (-9.9959, 23.5, -9.2344) (-10.9387, 23.5, -9.4368) (-12.019, 23.5, -9.6298) (-12.5398, 23.5, -9.1107) (-12.8725, 23.5, -8.455) (-12.3551, 23.5, -7.4872) (-11.8713, 23.5, -6.653) (-12.0731, 23.5, -6.1516) (-12.3602, 23.5, -5.6935) (-13.3194, 23.5, -5.5947) (-14.4065, 23.5, -5.4444) (-14.7414, 23.5, -4.7898) (-14.8552, 23.5, -4.0633) (-14.0641, 23.5, -3.3028) (-13.3462, 23.5, -2.659) (-13.3832, 23.5, -2.1197) (-13.5147, 23.5, -1.5954) (-14.3964, 23.5, -1.2049) (-15.3838, 23.5, -0.7261) (-15.5, 23.5, 0) (-15.3838, 23.5, 0.7261) (-14.3964, 23.5, 1.2049) (-13.5147, 23.5, 1.5954) (-13.3832, 23.5, 2.1197) (-13.3462, 23.5, 2.659) (-14.0641, 23.5, 3.3028) (-14.8552, 23.5, 4.0633) (-14.7414, 23.5, 4.7898) (-14.4065, 23.5, 5.4444) (-13.3194, 23.5, 5.5947) (-12.3602, 23.5, 5.6935) (-12.0731, 23.5, 6.1516) (-11.8713, 23.5, 6.653) (-12.3551, 23.5, 7.4872) (-12.8725, 23.5, 8.455) (-12.5398, 23.5, 9.1107) (-12.019, 23.5, 9.6298) (-10.9387, 23.5, 9.4368) (-9.9959, 23.5, 9.2344) (-9.5813, 23.5, 9.5813) (-9.2344, 23.5, 9.9959) (-9.4368, 23.5, 10.9387) (-9.6298, 23.5, 12.019) (-9.1107, 23.5, 12.5398) (-8.455, 23.5, 12.8725) (-7.4872, 23.5, 12.3551) (-6.653, 23.5, 11.8713) (-6.1516, 23.5, 12.0731) (-5.6935, 23.5, 12.3602) (-5.5947, 23.5, 13.3194) (-5.4444, 23.5, 14.4065) (-4.7898, 23.5, 14.7414) (-4.0633, 23.5, 14.8552) (-3.3028, 23.5, 14.0641) (-2.659, 23.5, 13.3462) (-2.1197, 23.5, 13.3832) (-1.5954, 23.5, 13.5147) (-1.2049, 23.5, 14.3964) (-0.7261, 23.5, 15.3838) (0, 23.5, 15.5) (0.7261, 23.5, 15.3838) (1.2049, 23.5, 14.3964) (1.5954, 23.5, 13.5147) (2.1197, 23.5, 13.3832) (2.659, 23.5, 13.3462) (3.3028, 23.5, 14.0641) (4.0633, 23.5, 14.8552) (4.7898, 23.5, 14.7414) (5.4444, 23.5, 14.4065) (5.5947, 23.5, 13.3194) (5.6935, 23.5, 12.3602) (6.1516, 23.5, 12.0731) (6.653, 23.5, 11.8713) (7.4872, 23.5, 12.3551) (8.455, 23.5, 12.8725) (9.1107, 23.5, 12.5398) (9.6298, 23.5, 12.019) (9.4368, 23.5, 10.9387) (9.2344, 23.5, 9.9959) (9.5813, 23.5, 9.5813) (9.9959, 23.5, 9.2344) (10.9387, 23.5, 9.4368) (12.019, 23.5, 9.6298) (12.5398, 23.5, 9.1107) (12.8725, 23.5, 8.455) (12.3551, 23.5, 7.4872) (11.8713, 23.5, 6.653) (12.0731, 23.5, 6.1516) (12.3602, 23.5, 5.6935) (13.3194, 23.5, 5.5947) (14.4065, 23.5, 5.4444) (14.7414, 23.5, 4.7898) (14.8552, 23.5, 4.0633) (14.0641, 23.5, 3.3028) (13.3462, 23.5, 2.659) (13.3832, 23.5, 2.1197) (13.5147, 23.5, 1.5954) (14.3964, 23.5, 1.2049) (15.3838, 23.5, 0.7261) (15.5, 23.5, 0) (15.3838, 23.5, -0.7261) (14.3964, 23.5, -1.2049) (13.5147, 23.5, -1.5954) (13.3832, 23.5, -2.1197) (13.3462, 23.5, -2.659) (14.0641, 23.5, -3.3028) (14.8552, 23.5, -4.0633) (14.7414, 23.5, -4.7898) (14.4065, 23.5, -5.4444) (13.3194, 23.5, -5.5947) (12.3602, 23.5, -5.6935) (12.0731, 23.5, -6.1516) (11.8713, 23.5, -6.653) (12.3551, 23.5, -7.4872) (12.8725, 23.5, -8.455) (12.5398, 23.5, -9.1107) (12.019, 23.5, -9.6298) (10.9387, 23.5, -9.4368) (9.9959, 23.5, -9.2344) (9.4368, 9.5, -10.9387) (9.2344, 9.5, -9.9959) (9.5813, 9.5, -9.5813) (9.9959, 9.5, -9.2344) (10.9387, 9.5, -9.4368) (12.3551, 9.5, -7.4872) (11.8713, 9.5, -6.653) (12.0731, 9.5, -6.1516) (12.3602, 9.5, -5.6935) (13.3194, 9.5, -5.5947) (14.0641, 9.5, -3.3028) (13.3462, 9.5, -2.659) (13.3832, 9.5, -2.1197) (13.5147, 9.5, -1.5954) (14.3964, 9.5, -1.2049) (14.3964, 9.5, 1.2049) (13.5147, 9.5, 1.5954) (13.3832, 9.5, 2.1197) (13.3462, 9.5, 2.659) (14.0641, 9.5, 3.3028) (13.3194, 9.5, 5.5947) (12.3602, 9.5, 5.6935) (12.0731, 9.5, 6.1516) (11.8713, 9.5, 6.653) (12.3551, 9.5, 7.4872) (10.9387, 9.5, 9.4368) (9.9959, 9.5, 9.2344) (9.5813, 9.5, 9.5813) (9.2344, 9.5, 9.9959) (9.4368, 9.5, 10.9387) (7.4872, 9.5, 12.3551) (6.653, 9.5, 11.8713) (6.1516, 9.5, 12.0731) (5.6935, 9.5, 12.3602) (5.5947, 9.5, 13.3194) (3.3028, 9.5, 14.0641) (2.659, 9.5, 13.3462) (2.1197, 9.5, 13.3832) (1.5954, 9.5, 13.5147) (1.2049, 9.5, 14.3964) (-1.2049, 9.5, 14.3964) (-1.5954, 9.5, 13.5147) (-2.1197, 9.5, 13.3832) (-2.659, 9.5, 13.3462) (-3.3028, 9.5, 14.0641) (-5.5947, 9.5, 13.3194) (-5.6935, 9.5, 12.3602) (-6.1516, 9.5, 12.0731) (-6.653, 9.5, 11.8713) (-7.4872, 9.5, 12.3551) (-9.4368, 9.5, 10.9387) (-9.2344, 9.5, 9.9959) (-9.5813, 9.5, 9.5813) (-9.9959, 9.5, 9.2344) (-10.9387, 9.5, 9.4368) (-12.3551, 9.5, 7.4872) (-11.8713, 9.5, 6.653) (-12.0731, 9.5, 6.1516) (-12.3602, 9.5, 5.6935) (-13.3194, 9.5, 5.5947) (-14.0641, 9.5, 3.3028) (-13.3462, 9.5, 2.659) (-13.3832, 9.5, 2.1197) (-13.5147, 9.5, 1.5954) (-14.3964, 9.5, 1.2049) (-14.3964, 9.5, -1.2049) (-13.5147, 9.5, -1.5954) (-13.3832, 9.5, -2.1197) (-13.3462, 9.5, -2.659) (-14.0641, 9.5, -3.3028) (-13.3194, 9.5, -5.5947) (-12.3602, 9.5, -5.6935) (-12.0731, 9.5, -6.1516) (-11.8713, 9.5, -6.653) (-12.3551, 9.5, -7.4872) (-10.9387, 9.5, -9.4368) (-9.9959, 9.5, -9.2344) (-9.5813, 9.5, -9.5813) (-9.2344, 9.5, -9.9959) (-9.4368, 9.5, -10.9387) (-7.4872, 9.5, -12.3551) (-6.653, 9.5, -11.8713) (-6.1516, 9.5, -12.0731) (-5.6935, 9.5, -12.3602) (-5.5947, 9.5, -13.3194) (-3.3028, 9.5, -14.0641) (-2.659, 9.5, -13.3462) (-2.1197, 9.5, -13.3832) (-1.5954, 9.5, -13.5147) (-1.2049, 9.5, -14.3964) (1.2049, 9.5, -14.3964) (1.5954, 9.5, -13.5147) (2.1197, 9.5, -13.3832) (2.659, 9.5, -13.3462) (3.3028, 9.5, -14.0641) (5.5947, 9.5, -13.3194) (5.6935, 9.5, -12.3602) (6.1516, 9.5, -12.0731) (6.653, 9.5, -11.8713) (7.4872, 9.5, -12.3551)
sketch "Sketch9" plane through (0, 25.5, 0) normal (0, 1, 0) x (1, 0, 0)
  circle A0 centre (0, 0) radius 1.5
  dimension "d43" = 3
  constraints: 1 centre point, 1 coincident
  measures "d43" diameter of A0
extrude "Extrusion9" cut sketch "Sketch9" against normal through all
sketch "Sketch10" plane through (0, 25.5, 0) normal (0, 1, 0) x (1, 0, 0)
  circle A0 centre (0, 0) radius 3
  dimension "d46" = 6
  constraints: 1 centre point, 1 coincident
  measures "d46" diameter of A0
extrude "Extrusion10" cut sketch "Sketch10" against normal blind 5
fillet "Fillet1" radius 0.25 1 edges at (-3, 25.5, 0)
sketch "Sketch11" plane through (0, -1.75, 0) normal (0, -1, 0) x (1, 0, 0)
  line L0 (0, -6.8705) -> (5.95, -3.4352) projected
  circle A0 centre (0, 0) radius 6.8705
  circle A1 centre (0, 0) radius 3.25 projected
  circle A2 centre (0, 0) radius 1.5 projected
  line L1 (4.95, -2.8579) -> (4.95, 2.8579) projected
  line L2 (4.95, 2.8579) -> (0, 5.7158) projected
  line L3 (0, 5.7158) -> (-4.95, 2.8579) projected
  line L4 (-4.95, 2.8579) -> (-4.95, -2.8579) projected
  line L5 (-4.95, -2.8579) -> (0, -5.7158) projected
  line L6 (0, -5.7158) -> (4.95, -2.8579) projected
  point P0 (0, -6.8705)
  constraints: 1 coincident, 3 other
extrude "Extrusion11" cut sketch "Sketch11" against normal up to surface (1.75 mm away) contours A0 L0 picked at (5.5902, 0)
body "Solid1"
